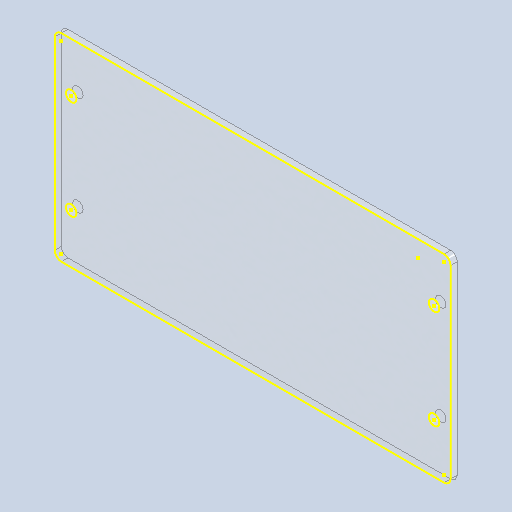
# Autodesk Inventor part: part4
Saved by Autodesk Inventor 2025.2 (Build 292293000, 293)
## iProperties
Created: 2025-02-28
Part Number: part4
Material: アクリル、クリア
Document SubType Name: Modeling
Designer: haruy
Density: 1.19 g/cm^3
Appearance: 透明 - クリア
Author: haruy
Autodesk Inventor part; units mm, degrees
ref_plane "YZ Plane" through (0, 0, 0) normal (1, 0, 0) x (0, 1, 0)
ref_plane "XZ Plane" through (0, 0, 0) normal (0, 1, 0) x (-1, 0, 0)
ref_plane "XY Plane" through (0, 0, 0) normal (0, 0, 1) x (1, 0, 0)
derived "oikon-Sketch-Base.ipt"
sketch "スケッチ2" plane through (0, 0, 0) normal (0, 0, 1) x (1, 0, 0)
  line L0 (0, 0) -> (-100, 0) projected
  line L1 (-100, 0) -> (-100, -50) projected
  line L2 (-100, -50) -> (0, -50) projected
  line L3 (0, -50) -> (0, 0) projected
  line L4 (0, -9) -> (-25.2, -9) projected
  line L5 (-25.2, -9) -> (-25.2, -17) projected
  line L6 (-25.2, -17) -> (0, -17) projected
  line L7 (0, -17) -> (0, -9) projected
  line L8 (0, -50) -> (10, -50) projected
  line L9 (10, -50) -> (10, 0) projected
  line L10 (10, 0) -> (0, 0) projected
  line L11 (0, 0) -> (0, -50) projected
  line L12 (-100, -50) -> (-110, -50) projected
  line L13 (-110, -50) -> (-110, 0) projected
  line L14 (-110, 0) -> (-100, 0) projected
  line L15 (-100, 0) -> (-100, -50) projected
  line L16 (-10.1, -7) -> (-15.1, -7) projected
  line L17 (-15.1, -7) -> (-15.1, -25.7) projected
  line L18 (-15.1, -25.7) -> (-10.1, -25.7) projected
  line L19 (-10.1, -25.7) -> (-10.1, -7) projected
  circle A0 centre (-5, -14) radius 1.6 projected
  line L20 (-12.6, -25.7) -> (-12.6, -7) projected
  circle A1 centre (-20.2, -14) radius 1.6 projected
  line L21 (-37.4, -9) -> (-62.6, -9) projected
  line L22 (-62.6, -9) -> (-62.6, -17) projected
  line L23 (-62.6, -17) -> (-37.4, -17) projected
  line L24 (-37.4, -17) -> (-37.4, -9) projected
  circle A2 centre (-42.4, -14) radius 1.6 projected
  circle A3 centre (-57.6, -14) radius 1.6 projected
  circle A4 centre (-79.8, -14) radius 1.6 projected
  circle A5 centre (-95, -14) radius 1.6 projected
  circle A6 centre (5, -10) radius 1.6 projected
  circle A7 centre (5, -40) radius 1.6 projected
  line L25 (-50, 0) -> (-50, -50) projected
  circle A8 centre (-105, -10) radius 1.6 projected
  circle A9 centre (-105, -40) radius 1.6 projected
  line L26 (-47.5, -6) -> (-52.5, -6) projected
  line L27 (-52.5, -6) -> (-52.5, -47.8) projected
  line L28 (-52.5, -47.8) -> (-47.5, -47.8) projected
  line L29 (-47.5, -47.8) -> (-47.5, -6) projected
  line L30 (-84.9, -7) -> (-89.9, -7) projected
  line L31 (-89.9, -7) -> (-89.9, -36.3712) projected
  line L32 (-89.9, -36.3712) -> (-84.9, -36.3712) projected
  line L33 (-84.9, -36.3712) -> (-84.9, -7) projected
  line L34 (10, 0) -> (-110, 0) projected
  line L35 (-110, 0) -> (-110, 5) projected
  line L36 (-110, 5) -> (10, 5) projected
  line L37 (10, 5) -> (10, 0) projected
  line L38 (10, -50) -> (-110, -50) projected
  line L39 (-110, -50) -> (-110, -55) projected
  line L40 (-110, -55) -> (10, -55) projected
  line L41 (10, -55) -> (10, -50) projected
  circle A10 centre (-5, -5) radius 1.6 projected
  line L42 (10, -25) -> (-100, -25) projected
  circle A11 centre (-5, -45) radius 1.6 projected
  circle A12 centre (-95, -45) radius 1.6 projected
  circle A13 centre (-95, -5) radius 1.6 projected
  line L43 (-15.2, -6.9) -> (-10, -6.9) projected
  line L44 (-10, -6.9) -> (-10, -25.8) projected
  line L45 (-10, -25.8) -> (-15.2, -25.8) projected
  line L46 (-15.2, -25.8) -> (-15.2, -6.9) projected
  line L47 (-9.6, -47.8) -> (-15.6, -47.8) projected
  line L48 (-15.6, -47.8) -> (-15.6, -25.8) projected
  line L49 (-15.6, -25.8) -> (-9.6, -25.8) projected
  line L50 (-9.6, -25.8) -> (-9.6, -47.8) projected
  line L51 (-53, -47.8) -> (-53, -25.8) projected
  line L52 (-47, -47.8) -> (-53, -47.8) projected
  line L53 (-47, -25.8) -> (-47, -47.8) projected
  line L54 (-53, -25.8) -> (-47, -25.8) projected
  line L55 (-47.4, -6.9) -> (-47.4, -25.8) projected
  line L56 (-52.6, -25.8) -> (-52.6, -6.9) projected
  line L57 (-52.6, -6.9) -> (-47.4, -6.9) projected
  line L58 (-90.4, -47.8) -> (-90.4, -25.8) projected
  line L59 (-84.4, -47.8) -> (-90.4, -47.8) projected
  line L60 (-84.4, -25.8) -> (-84.4, -47.8) projected
  line L61 (-90.4, -25.8) -> (-84.4, -25.8) projected
  line L62 (-84.8, -6.9) -> (-84.8, -25.8) projected
  line L63 (-90, -25.8) -> (-90, -6.9) projected
  line L64 (-90, -6.9) -> (-84.8, -6.9) projected
  line L65 (-11.6, -25.8) -> (-13.6, -25.8) projected
  line L66 (-13.6, -25.8) -> (-13.6, -6.9) projected
  line L67 (-13.6, -6.9) -> (-11.6, -6.9) projected
  line L68 (-11.6, -6.9) -> (-11.6, -25.8) projected
  line L69 (-11.5, -25.9) -> (-13.7, -25.9) projected
  line L70 (-13.7, -25.9) -> (-13.7, -6.8) projected
  line L71 (-13.7, -6.8) -> (-11.5, -6.8) projected
  line L72 (-11.5, -6.8) -> (-11.5, -25.9) projected
  line L73 (-48.9, -25.9) -> (-51.1, -25.9) projected
  line L74 (-48.9, -6.8) -> (-48.9, -25.9) projected
  line L75 (-51.1, -25.9) -> (-51.1, -6.8) projected
  line L76 (-51, -25.8) -> (-51, -6.9) projected
  line L77 (-49, -6.9) -> (-49, -25.8) projected
  line L78 (-51.1, -6.8) -> (-48.9, -6.8) projected
  line L79 (-86.3, -25.9) -> (-88.5, -25.9) projected
  line L80 (-86.3, -6.8) -> (-86.3, -25.9) projected
  line L81 (-88.5, -25.9) -> (-88.5, -6.8) projected
  line L82 (-88.4, -25.8) -> (-88.4, -6.9) projected
  line L83 (-86.4, -6.9) -> (-86.4, -25.8) projected
  line L84 (-88.5, -6.8) -> (-86.3, -6.8) projected
  point P0 (-84.8, -25.8)
  point P1 (-84.9, -25.8)
  point P2 (-89.9, -25.8)
  point P3 (-90, -25.8)
  point P4 (-52.5, -9)
  point P5 (-52.6, -9)
  point P6 (-47.4, -9)
  point P7 (-47.5, -9)
  point P8 (-52.5, -17)
  point P9 (-52.5, -47.8)
  point P10 (-52.6, -25.8)
  point P11 (-52.6, -17)
  point P12 (-47.5, -17)
  point P13 (-47.4, -17)
  point P14 (-47.4, -25.8)
  point P15 (-52.5, -6.9)
  point P16 (-47.5, -6.9)
  constraints: 3 horizontal
extrude "押し出し1" add sketch "スケッチ2" along normal blind 2 contours L3 L4 L44 L43 L72 L71 L70 L46 L5 L6 L42 L55 L23 L24 L21 L57 L29 L26 L25 L0 | L10 L9 L42 L3 | L0 L14 L35 L36 L37 L10 | L25 L26 L27 L57 L56 L21 L22 L23 L42 L62 L64 L80 L84 L81 L63 L1 L0 | L3 L6 L44 L4 | L1 L12 L13 L14 | L26 L29 L57 L74 L78 L25 | L25 L78 L75 L57 L27 L26 | L3 L42 L44 L6 | L44 L6 L19 L4 | L4 L19 L16 L72 L43 L44 | L9 L8 L3 L42 | L42 L63 L61 L58 L59 L60 L62 L56 L54 L51 L52 L28 L25 L2 L1 | L78 L74 L57 L25 | L25 L57 L75 L78 | L3 L2 L25 L28 L52 L53 L54 L55 L42 L46 L49 L48 L47 L50 L44 | L44 L42 L19 L6 | L19 L6 L72 L4 | L4 L72 L16 L19 | L41 L40 L39 L12 L2 L8 | L63 L64 L81 L30 L31 L42 | L42 L31 L61 L63 | L57 L77 L21 L25 | L25 L21 L76 L57 | L57 L55 L21 L29 | L29 L21 L74 L57 | L57 L75 L21 L27 | L27 L21 L56 L57 | L44 L45 L72 L18 L19 L42 | L19 L42 L72 L6 | L72 L6 L68 L4 | L4 L68 L16 L72 | L72 L16 L68 L43 | L43 L70 L71 L72 | L42 L81 L61 L31 | L31 L30 L81 L42 | L61 L31 L32 L33 L60 L59 L58 | L25 L23 L76 L21 | L21 L77 L23 L25 | L76 L21 L75 L57 | L57 L74 L21 L77 | L29 L23 L74 L21 | L21 L55 L23 L29 | L27 L23 L56 L21 | L21 L75 L23 L27 | L19 L18 L72 L42 | L49 L50 L47 L48 L45 L70 L69 L72 | L72 L42 L68 L6 | L68 L6 L20 L4 | L4 L20 L16 L68 | L68 L16 L66 L43 | L28 L27 L54 L75 L73 L25 | L25 L73 L74 L54 L29 L28 | L61 L81 L79 L80 L33 L32 L31 | L81 L30 L82 L42 | L42 L82 L61 L81 | L81 L84 L80 L64 | L64 L82 L30 L81 | L21 L74 L23 L77 | L76 L23 L75 L21 | L25 L42 L76 L23 | L23 L77 L42 L25 | L21 L24 L23 L55 | L29 L42 L74 L23 | L23 L55 L42 L29 | L56 L23 L22 L21 | L27 L42 L56 L23 | L23 L75 L42 L27 | L72 L18 L68 L42 | L72 L69 L70 L45 | L45 L68 L18 L72 | L68 L42 L20 L6 | L20 L6 L66 L4 | L4 L66 L16 L20 | L66 L16 L70 L43 | L73 L75 L54 L25 | L25 L54 L74 L73 | L52 L51 L54 L27 | L29 L54 L53 L52 | L61 L80 L79 L81 | L82 L30 L83 L42 | L42 L83 L61 L82 | L64 L83 L30 L82 | L23 L74 L42 L77 | L76 L42 L75 L23 | L42 L77 L54 L25 | L25 L54 L76 L42 | L42 L55 L54 L29 | L29 L54 L74 L42 | L42 L75 L54 L27 | L27 L54 L56 L42 | L68 L18 L20 L42 | L45 L66 L18 L68 | L20 L42 L66 L6 | L66 L6 L70 L4 | L4 L70 L16 L66 | L70 L16 L17 L4 L46 L43 | L83 L30 L80 L42 | L42 L80 L61 L83 | L64 L80 L30 L83 | L42 L74 L54 L77 | L76 L54 L75 L42 | L20 L18 L66 L42 | L45 L70 L18 L66 | L66 L42 L70 L6 | L70 L6 L17 L4 | L4 L17 L16 L70 | L61 L80 L42 L33 | L33 L42 L62 L61 | L80 L30 L33 L42 | L64 L62 L42 L33 L30 L80 | L46 L6 L17 L42 | L42 L17 L18 L70 L45 L46 | L66 L18 L70 L42 | L70 L42 L17 L6 | L17 L6 L46 L4 | L46 L6 L5 L4 | L42 L70 L18 L17 | A0 | A1 | A2 | A3 | A4 | A5 | A10 | A11 | A12 | A13
fillet "フィレット1" radius 2 4 edges at (10, 5, 1) (10, -55, 1) (-110, -55, 1) (-110, 5, 1)
sketch "スケッチ3" plane through (-108, -55, 2) normal (0, 0, 1) x (1, 0, 0)
  arc A0 (0, 60) -> (-2, 58) centre (0, 58) ccw projected
  line L0 (-2, 58) -> (-2, 2) projected
  arc A1 (-2, 2) -> (0, 0) centre (0, 2) ccw projected
  line L1 (0, 0) -> (116, 0) projected
  arc A2 (116, 0) -> (118, 2) centre (116, 2) ccw projected
  line L2 (118, 2) -> (118, 58) projected
  arc A3 (118, 58) -> (116, 60) centre (116, 58) ccw projected
  line L3 (116, 60) -> (0, 60) projected
  circle A4 centre (113, 15) radius 1.6 projected
  circle A5 centre (3, 45) radius 1.6 projected
  circle A6 centre (113, 45) radius 1.6 projected
  circle A7 centre (3, 15) radius 1.6 projected
  point P0 (108, 55)
